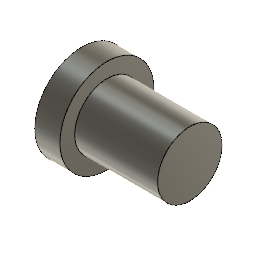
103_CCTV_Lens_f2.8_f#1.4 v1 (Autodesk Fusion 360 design; units mm, degrees)
Autodesk Fusion 360 part; units mm, degrees
sketch "Sketch1" plane through (0, 0, 0) normal (0, 1, 0) x (1, 0, 0)
  line L0 (0, 0) -> (-15.4, 0)
  line L1 (0, 0) -> (0, 6)
  line L2 (0, 6) -> (-15.4, 6)
  line L3 (-15.4, 6) -> (-15.4, 8.75)
  line L4 (-15.4, 8.75) -> (-20.1, 8.75)
  arc A0 (-20.1, 8.75) -> (-23, 0) centre (-9.8582, 0.5) ccw
  line L5 (-23, 0) -> (-15.4, 0)
  dimension "d1" = 15.4
  dimension "d2" = 6
  dimension "d3" = 15.4
  dimension "d4" = 2.75
  dimension "d5" = 90
  dimension "d6" = 4.7
  constraint horizontal L0
  constraint coincident L0.start L1.start
  constraint vertical L1
  constraint horizontal L2
  constraint perpendicular L2 L3
  constraint parallel L0 L5
  measures "d1" distance of L0.start L0.end
  measures "d2" distance of L0.start L1.end
  measures "d3" distance of L1.end L2.end
  measures "d4" distance of L2.end L3.end
  measures "d5" angle of L3 L4
  measures "d6" distance of L3.end L4.end
revolve "Revolve1" add sketch "Sketch1" angle 360 about axis through (0, 0, 0) along (-1, 0, 0)
equation "d2 = ( 12 / 2 ) * 1 mm"
equation "d4 = ( 17.5 mm - 12 mm ) / 2"
